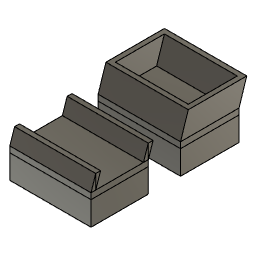
halterung v4 (Autodesk Fusion 360 design; units mm, degrees)
Autodesk Fusion 360 part; units mm, degrees
sketch "Skizze15" plane through (0, 0, 0) normal (0, 0, 1) x (1, 0, 0)
  line L0 (34, 24) -> (-34, 24)
  line L1 (-34, 24) -> (-34, -24)
  line L2 (-34, -24) -> (34, -24)
  line L3 (34, -24) -> (34, 24)
  line L4 (34, 24) -> (-34, -24) construction
  line L5 (-34, 24) -> (34, -24) construction
  dimension "d68" = 68
  dimension "d69" = 48
  constraint perpendicular L0 L1
  constraint parallel L0 L2
  constraint parallel L1 L3
  constraint horizontal L0
  constraint coincident L4 origin
  constraint coincident L5 origin
  measures "d68" distance of L1.end L2.end
  measures "d69" distance of L0.end L1.end
extrude "Extrusion21" add sketch "Skizze15" along normal blind 20 makes body 1
extrude "Extrusion22" add 1 faces at (11.3333, -8, 20) along direction (0, 0, 1) blind 5 separate body on bodies 1 makes body 2
sketch "Skizze16" plane through (0, 0, 0) normal (0, 0, -1) x (1, 0, 0)
  line L0 (34, -24) -> (34, 24)
  line L1 (34, 24) -> (-34, 24)
  line L2 (-34, 24) -> (-34, -24)
  line L3 (-34, -24) -> (34, -24)
  line L4 (-30, 20) -> (30, 20)
  line L5 (30, 20) -> (30, -20)
  line L6 (30, -20) -> (-30, -20)
  line L7 (-30, -20) -> (-30, 20)
  dimension "d74" = 60
  dimension "d75" = 40
  constraint horizontal L4
  constraint vertical L5
  constraint horizontal L6
  constraint vertical L7
  measures "d74" distance of L4.start L4.end
  measures "d75" distance of L4.start L6.end
extrude "Extrusion23" cut sketch "Skizze16" against normal blind 20 contours L4 L5 L6 L7 bodies 1
sketch "Skizze17" plane through (0, 0, 25) normal (0, 0, 1) x (-1, 0, 0)
  line L0 (-34, 24) -> (-34, -24)
  line L1 (-34, -24) -> (34, -24)
  line L2 (34, -24) -> (34, 24)
  line L3 (34, 24) -> (-34, 24)
  line L4 (30, -20) -> (-30, -20)
  line L5 (-30, -20) -> (-30, 20)
  line L6 (-30, 20) -> (30, 20)
  line L7 (30, 20) -> (30, -20)
  line L8 (-34, -20) -> (-30, -20)
  line L9 (-30, -20) -> (-30, 20)
  line L10 (-30, 20) -> (-34, 20)
  line L11 (-34, 20) -> (-34, -20)
  line L12 (30, -20) -> (34, -20)
  line L13 (34, -20) -> (34, 20)
  line L14 (34, 20) -> (30, 20)
  line L15 (30, 20) -> (30, -20)
  line L16 (34, 20) -> (-34, 20)
  line L17 (-34, 20) -> (-34, 24)
  line L18 (-34, 24) -> (34, 24)
  line L19 (34, 24) -> (34, 20)
  line L20 (-34, -24) -> (34, -24)
  line L21 (34, -24) -> (34, -20)
  line L22 (34, -20) -> (-34, -20)
  line L23 (-34, -20) -> (-34, -24)
  point P0 (30, -20)
  dimension "d78" = 60
  dimension "d79" = 40
  constraint horizontal L4
  constraint vertical L5
  constraint horizontal L6
  constraint vertical L7
  constraint coincident P0 L4.start
  constraint horizontal L8
  constraint vertical L9
  constraint horizontal L10
  constraint vertical L11
  constraint coincident L0 L8.start
  constraint horizontal L12
  constraint vertical L13
  constraint horizontal L14
  constraint vertical L15
  constraint coincident L2 L13.end
  constraint horizontal L16
  constraint vertical L17
  constraint horizontal L18
  constraint vertical L19
  constraint coincident L0.start L3.end
  constraint horizontal L20
  constraint vertical L21
  constraint horizontal L22
  constraint vertical L23
  constraint coincident L0.end L1.start
  measures "d78" distance of P0 L4.end
  measures "d79" distance of P0 L6.end
extrude "Extrusion24" add sketch "Skizze17" along normal blind 12 separate body contours L0 L2 L3 L6 L10 L14 L16 L17 L18 L19 | L0 L1 L2 L4 L8 L12 L20 L21 L22 L23 makes body 3 at (11.3333, 24, 29) makes body 4 at (-11.3333, -24, 29)
chamfer "Fase5" distance 4 distance2 12 2 edges at (0, 20, 37) (0, -24, 37) measured on face at (11.3333, 22.6667, 37) measured on face at (11.3333, -22.6667, 37) on bodies 3 4
extrude "Extrusion25" add 1 faces at (-11.3333, -20, 29) along direction (0, 1, 0) blind 4 separate body on bodies 4 makes body 5
extrude "Extrusion26" add 1 faces at (11.3333, 24, 29) along direction (0, 1, 0) blind 4 separate body on bodies 3 makes body 6
chamfer "Fase6" distance 12 distance2 4 1 edges at (0, -16, 25) measured on face at (-11.3333, -16, 29) on bodies 5
chamfer "Fase7" distance 12 distance2 4 1 edges at (0, 28, 25) measured on face at (11.3333, 28, 29) on bodies 6
sketch "Skizze18" plane through (0, 0, 0) normal (0, 0, 1) x (1, 0, 0)
  line L0 (34.5, 50.5) -> (-34.5, 50.5)
  line L1 (-34.5, 50.5) -> (-34.5, 99.5)
  line L2 (-34.5, 99.5) -> (34.5, 99.5)
  line L3 (34.5, 99.5) -> (34.5, 50.5)
  line L4 (34.5, 50.5) -> (-34.5, 99.5) construction
  line L5 (-34.5, 50.5) -> (34.5, 99.5) construction
  point P0 (0, 75)
  dimension "d92" = 69
  dimension "d93" = 49
  constraint perpendicular L0 L1
  constraint parallel L0 L2
  constraint parallel L1 L3
  constraint horizontal L0
  constraint coincident L4 P0
  constraint coincident L5 P0
  measures "d92" distance of L1.end L2.end
  measures "d93" distance of L0.end L1.end
extrude "Extrusion27" add sketch "Skizze18" along normal blind 20 separate body makes body 7
sketch "Skizze19" plane through (0, 0, 20) normal (0, 0, 1) x (-1, 0, 0)
  line L0 (-34.5, -99.5) -> (34.5, -99.5)
  line L1 (34.5, -99.5) -> (34.5, -50.5)
  line L2 (34.5, -50.5) -> (-34.5, -50.5)
  line L3 (-34.5, -50.5) -> (-34.5, -99.5)
  line L4 (-30.5, -95.5) -> (30.5, -95.5)
  line L5 (30.5, -95.5) -> (30.5, -54.5)
  line L6 (30.5, -54.5) -> (-30.5, -54.5)
  line L7 (-30.5, -54.5) -> (-30.5, -95.5)
  line L8 (-30.5, -95.5) -> (30.5, -54.5) construction
  line L9 (30.5, -95.5) -> (-30.5, -54.5) construction
  point P0 (0, -75)
  dimension "d96" = 61
  dimension "d97" = 41
  constraint perpendicular L4 L5
  constraint parallel L4 L6
  constraint parallel L5 L7
  constraint horizontal L4
  constraint coincident L8 P0
  constraint coincident L9 P0
  measures "d96" distance of L5.end L6.end
  measures "d97" distance of L4.end L5.end
extrude "Extrusion28" cut sketch "Skizze19" against normal blind 20 contours L4 L5 L6 L7 bodies 7
extrude "Extrusion29" add 1 faces at (-10.1667, 98.1667, 20) along direction (0, 0, 1) blind 5 separate body on bodies 7 makes body 8
extrude "Extrusion30" add 1 faces at (30.5, 68.1667, 23.3333) along direction (-1, 0, 0) blind 61 separate body on bodies 8 makes body 9
extrude "Extrusion31" add 1 faces at (-10.1667, 98.1667, 25) along direction (0, 0, 1) blind 20 separate body on bodies 8 makes body 10
draft "Entwurf2" angle -18 neutral plane through (30.5, 54.5, 25) pull (0, 0, 1) 1 faces at (-11.5, 99.5, 31.6667) on bodies 10
draft "Entwurf3" angle -18 neutral plane through (30.5, 54.5, 25) pull (0, 0, 1) 1 faces at (-10.1667, 54.5, 31.6667) on bodies 10
draft "Entwurf4" angle 18 neutral plane through (30.5, 54.5, 25) pull (0, 0, 1) 1 faces at (11.5, 50.5, 31.6667) on bodies 10
draft "Entwurf5" angle 18 neutral plane through (30.5, 54.5, 25) pull (0, 0, 1) 1 faces at (10.1667, 95.5, 31.6667) on bodies 10
